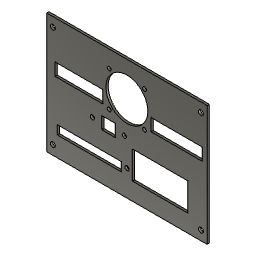
CNC_Control_Panels (Autodesk Fusion 360 design; units mm, degrees)
Autodesk Fusion 360 part; units mm, degrees
sketch "Sketch1" plane through (0, 0, 0) normal (0, 1, 0) x (1, 0, 0)
  line L0 (0, 0) -> (145.5, 0)
  line L1 (145.5, 0) -> (145.5, -109)
  line L2 (145.5, -109) -> (0, -109)
  line L3 (0, -109) -> (0, 0)
  line L4 (5.65, -100.6) -> (139.85, -100.6) construction
  line L5 (139.85, -100.6) -> (139.85, -8.4) construction
  line L6 (139.85, -8.4) -> (5.65, -8.4) construction
  line L7 (5.65, -8.4) -> (5.65, -100.6) construction
  circle A0 centre (5.65, -100.6) radius 2.25
  circle A1 centre (139.85, -100.6) radius 2.25
  circle A2 centre (139.85, -8.4) radius 2.25
  circle A3 centre (5.65, -8.4) radius 2.25
  line L8 (72.75, -109) -> (72.75, 0) construction
  line L9 (0, -54.5) -> (145.5, -54.5) construction
  line L10 (77.7, -15.8) -> (128, -15.8)
  line L11 (128, -15.8) -> (128, -41.1)
  line L12 (128, -41.1) -> (77.7, -41.1)
  line L13 (77.7, -41.1) -> (77.7, -15.8)
  line L14 (9.7, -26.1) -> (67.7, -26.1)
  line L15 (67.7, -26.1) -> (67.7, -18)
  line L16 (67.7, -18) -> (9.7, -18)
  line L17 (9.7, -18) -> (9.7, -26.1)
  line L18 (7.6, -74.3) -> (50.9, -74.3)
  line L19 (50.9, -74.3) -> (50.9, -63)
  line L20 (50.9, -63) -> (7.6, -63)
  line L21 (7.6, -63) -> (7.6, -74.3)
  line L22 (94.7, -74.2) -> (141.1, -74.2)
  line L23 (141.1, -74.2) -> (141.1, -63)
  line L24 (141.1, -63) -> (94.7, -63)
  line L25 (94.7, -63) -> (94.7, -74.2)
  circle A4 centre (72.75, -77.6) radius 19
  circle A5 centre (72.85, -23.45) radius 1.95
  line L26 (72.85, -25.4) -> (72.85, -21.5) construction
  line L27 (70.9, -23.45) -> (74.8, -23.45) construction
  line L28 (56.75, -93.6) -> (88.75, -93.6) construction
  line L29 (88.75, -93.6) -> (88.75, -61.6) construction
  line L30 (88.75, -61.6) -> (56.75, -61.6) construction
  line L31 (56.75, -61.6) -> (56.75, -93.6) construction
  line L32 (53.75, -77.6) -> (91.75, -77.6) construction
  circle A6 centre (56.75, -93.6) radius 1.75
  circle A7 centre (88.75, -93.6) radius 1.75
  circle A8 centre (56.75, -61.6) radius 1.75
  circle A9 centre (88.75, -61.6) radius 1.75
  line L33 (41.5, -47.8) -> (70.5, -47.8) construction
  circle A10 centre (70.5, -47.8) radius 1.9
  circle A11 centre (41.5, -47.8) radius 1.9
  line L34 (49.9, -53.4) -> (62.1, -53.4)
  line L35 (62.1, -53.4) -> (62.1, -42.2)
  line L36 (62.1, -42.2) -> (49.9, -42.2)
  line L37 (49.9, -42.2) -> (49.9, -53.4)
  line L38 (56, -53.4) -> (56, -42.2) construction
  point P0 (72.75, -96.6)
  dimension "d1" = 145.5
  dimension "d2" = 109
  dimension "d5" = 134.2
  dimension "d6" = 4.5
  dimension "d7" = 92.2
  dimension "d10" = 50.3
  dimension "d11" = 25.3
  dimension "d12" = 11.2
  dimension "d13" = 46.4
  dimension "d14" = 43.3
  dimension "d15" = 11.3
  dimension "d16" = 8.1
  dimension "d17" = 58
  dimension "d18" = 18
  dimension "d19" = 63
  dimension "d20" = 15.8
  dimension "d21" = 63
  dimension "d22" = 4.4
  dimension "d23" = 17.5
  dimension "d24" = 9.7
  dimension "d25" = 7.6
  dimension "d26" = 25.4
  dimension "d27" = 21.5
  dimension "d28" = 74.8
  dimension "d29" = 38
  dimension "d30" = 12.4
  dimension "d31" = 32
  dimension "d32" = 3.5
  dimension "d33" = 6.7
  dimension "d34" = 29
  dimension "d35" = 3.8
  dimension "d36" = 11.2
  dimension "d37" = 12.2
  dimension "d38" = 56
  constraint horizontal L0
  constraint vertical L1
  constraint horizontal L2
  constraint vertical L3
  constraint coincident L0.start L3.end
  constraint horizontal L4
  constraint vertical L5
  constraint horizontal L6
  constraint vertical L7
  constraint coincident L4.start L7.end
  constraint coincident L4.end L5.start
  constraint coincident L5.end L6.start
  constraint coincident L6.end L7.start
  constraint equal A0 A3
  constraint equal A2 A3
  constraint equal A1 A2
  constraint midpoint L2 L8.start
  constraint midpoint L0 L8.end
  constraint midpoint L3 L9.start
  constraint midpoint L1 L9.end
  constraint symmetric L4.start L4.end L8
  constraint symmetric L4.start L6.end L9
  constraint horizontal L10
  constraint vertical L11
  constraint horizontal L12
  constraint vertical L13
  constraint horizontal L14
  constraint vertical L15
  constraint horizontal L16
  constraint vertical L17
  constraint horizontal L18
  constraint vertical L19
  constraint horizontal L20
  constraint vertical L21
  constraint horizontal L22
  constraint vertical L23
  constraint horizontal L24
  constraint vertical L25
  constraint coincident A5 L26.start
  constraint coincident A5 L26.end
  constraint perpendicular L14 L26
  constraint coincident A5.centre L26
  constraint coincident A5 L27.start
  constraint coincident A5 L27.end
  constraint perpendicular L13 L27
  constraint coincident A5.centre L27
  constraint coincident L8 A4.centre
  constraint coincident A4 P0
  constraint coincident L8 P0
  constraint horizontal L28
  constraint vertical L29
  constraint horizontal L30
  constraint vertical L31
  constraint coincident A4 L32.start
  constraint coincident A4 L32.end
  constraint perpendicular L29 L32
  constraint coincident A4.centre L32
  constraint symmetric L28.start L30.end L32
  constraint symmetric L8 L28.start L28.end
  constraint equal L28 L31
  constraint coincident L28.start L31.end
  constraint coincident L28.end L29.start
  constraint coincident L30.end L31.start
  constraint coincident L29.end L30.start
  constraint equal A8 A9
  constraint equal A6 A8
  constraint equal A6 A7
  constraint horizontal L33
  constraint coincident L33.end A10.centre
  constraint coincident L33.start A11.centre
  constraint horizontal L34
  constraint vertical L35
  constraint horizontal L36
  constraint vertical L37
  constraint symmetric L33 L34.end L35.end
  constraint midpoint L34 L38.start
  constraint midpoint L36 L38.end
  constraint symmetric L33.end L33.start L38
  constraint equal A10 A11
  measures "d1" distance of L0.start L0.end
  measures "d2" distance of L0.start L2.end
  measures "d5" distance of L4.start L4.end
  measures "d6" diameter of A1
  measures "d7" distance of L4.end L5.end
  measures "d10" distance of L10.start L10.end
  measures "d11" distance of L10.end L11.end
  measures "d12" distance of L22.end L23.end
  measures "d13" distance of L23.end L24.end
  measures "d14" distance of L19.end L20.end
  measures "d15" distance of L18.start L20.end
  measures "d16" distance of L14.start L16.end
  measures "d17" distance of L15.end L16.end
  measures "d18" vertical distance of L0.start L16.end
  measures "d19" vertical distance of L0.start L20.end
  measures "d20" vertical distance of L0.end L10.end
  measures "d21" vertical distance of L0.end L23.end
  measures "d22" distance of L1 L22.end
  measures "d23" horizontal distance of L0.end L10.end
  measures "d24" horizontal distance of L0.start L16.end
  measures "d25" horizontal distance of L0.start L20.end
  measures "d26" distance of L0 L26.start
  measures "d27" distance of L0 L26.end
  measures "d28" horizontal distance of L0.start L27.end
  measures "d29" diameter of A4
  measures "d30" distance of L8.start P0
  measures "d31" distance of L28.start L28.end
  measures "d32" diameter of A6
  measures "d33" vertical distance of L12.end L33.end
  measures "d34" distance of L33.start L33.end
  measures "d35" diameter of A10
  measures "d36" distance of L34.start L36.end
  measures "d37" distance of L35.end L36.end
  measures "d38" horizontal distance of L9.start L38.start
extrude "Extrude1" add sketch "Sketch1" along normal blind 1.8 contours L0 L1 L2 L3 | L10 L11 L12 L13 | L14 L15 L16 L17 | L18 L19 L20 L21 | L22 L23 L24 L25 | A4 | A5 | A6 | A7 | A8 | A9 | A10 | A11 | L34 L35 L36 L37 makes body 1
extrude "Extrude2" add sketch "Sketch1" along normal blind 2 separate body makes body 2
hidden bodies 1
named bodies: "CNC_Control_Panel_top", "CNC_Control_Panel_bot"
